la1 (Autodesk Fusion 360 design; units mm, degrees)
Autodesk Fusion 360 part; units mm, degrees
sketch "Sketch1" plane through (0, 0, 0) normal (0, 1, 0) x (1, 0, 0)
  line L0 (0, 0) -> (120.5, 0)
  line L1 (120.5, 0) -> (120.5, -70.5)
  line L2 (120.5, -70.5) -> (0, -70.5)
  line L3 (0, -70.5) -> (0, 0)
  dimension "d1" = 120.5
  dimension "d2" = 70.5
  constraint horizontal L0
  constraint vertical L1
  constraint horizontal L2
  constraint vertical L3
  constraint coincident L0.start L3.end
  measures "d1" distance of L0.start L0.end
  measures "d2" distance of L0.start L2.end
extrude "Extrude1" add sketch "Sketch1" along normal blind 1.6
component "pcb" placed x (1, 0, 0) y (0, 1, 0) z (0, 0, 1) at (0, 0, 0)
